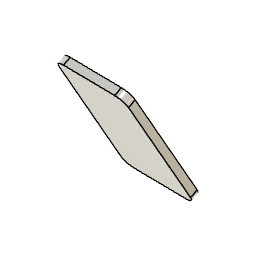
Phone Stand (Assembly) (Autodesk Fusion 360 archive; units mm, degrees)
design "Phone"
part number: 2026-06-04-19-47-22-060
Autodesk Fusion 360 part; units mm, degrees
sketch "Sketch1" plane through (0, 0, 0) normal (0, 0, 1) x (1, 0, 0)
  line L0 (0, 50) -> (-75, 50)
  line L1 (-75, 50) -> (-75, 205)
  line L2 (-75, 205) -> (0, 205)
  line L3 (0, 205) -> (0, 50)
  dimension "d1" = 75
  dimension "d2" = 155
  constraint horizontal L0
  constraint vertical L1
  constraint horizontal L2
  constraint vertical L3
  measures "d1" distance of L0.start L0.end
  measures "d2" distance of L0.start L2.end
extrude "Extrude1" add sketch "Sketch1" along normal blind 8
fillet "Fillet1" radius 10 1 edges at (0, 205, 4)
fillet "Fillet2" radius 10 1 edges at (-75, 205, 4)
fillet "Fillet3" radius 10 1 edges at (0, 50, 4)
fillet "Fillet4" radius 10 1 edges at (-75, 50, 4)
move_body "Move1" bodies 1 to x (0.996195, 0, -0.087156) y (-0.075479, 0.5, -0.86273) z (0.043578, 0.866025, 0.498097) at (214.0312, -116.6375, 222.5063)
move_body "Move2" bodies 1 to x (0.996202, -0.043268, 0.075562) y (0.043556, 0.999049, -0.002157) z (-0.075396, 0.00544, 0.997139) at (-105.4138, 10.2021, -14.7278)
move_body "Move3" bodies 1 to x (0.999848, 0.008699, -0.015111) y (-0.008687, 0.999962, 0.000826) z (0.015118, -0.000695, 0.999885) at (-2.1353, -0.3577, 0.8088)
move_body "Move4" bodies 1 to x (0.996197, 0.075622, 0.043275) y (-0.075527, 0.997136, -0.003823) z (-0.04344, 0.00054, 0.999056) at (2.0977, -3.783, -2.1098)
move_body "Move5" bodies 1 to x (0.99863, -0.045434, -0.025975) y (0.045426, 0.998967, -0.000894) z (0.025989, -0.000287, 0.999662) at (-0.665, 2.7758, 1.592)

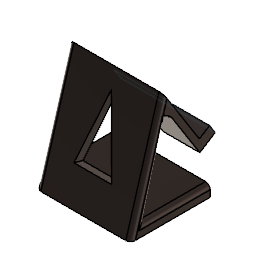
design "Phone Stand"
part number: 2026-06-02-13-47-00-270
Autodesk Fusion 360 part; units mm, degrees
sketch "Sketch1" plane through (0, 0, 0) normal (1, 0, 0) x (0, 1, 0)
  line L0 (0, 0) -> (-70, 0)
  line L1 (-70, 0) -> (-45.7841, 89.4173)
  line L2 (-45.7841, 89.4173) -> (-11.0619, 34.4149)
  line L3 (-11.0619, 34.4149) -> (5.2441, 44.7086)
  line L4 (5.2441, 44.7086) -> (-2.9089, 57.6236)
  line L5 (-2.9089, 57.6236) -> (-7.2276, 54.8973)
  line L6 (-7.2276, 54.8973) -> (-5.0683, 51.4767)
  line L7 (-5.0683, 51.4767) -> (-11.5885, 47.3606)
  line L8 (-11.5885, 47.3606) -> (-49.383, 107.2298)
  line L9 (-49.383, 107.2298) -> (-84.5009, -11.9838)
  line L10 (-84.5009, -11.9838) -> (0, -11.9838)
  line L11 (0, -11.9838) -> (0, 2.7655)
  constraint coincident L0.start origin
  constraint horizontal L0
  constraint perpendicular L2 L3
  constraint perpendicular L3 L4
  constraint perpendicular L4 L5
  constraint perpendicular L5 L6
  constraint perpendicular L4 L7
  constraint perpendicular L7 L8
  constraint horizontal L10
  constraint perpendicular L0 L11
extrude "Extrude1" add sketch "Sketch1" along normal blind 100
fillet "Fillet1" radius 2 2 edges at (50, -7.2276, 54.8973) (50, -2.9089, 57.6236)
sketch "Sketch2" plane through (0, 23.931, 15.1073) normal (0, 0.845601, 0.533815) x (-1, 0, 0)
  line L0 (0, 48.2794) -> (-100, 48.2794)
  line L1 (-100, 48.2794) -> (-100, 35.0063)
  line L2 (-100, 35.0063) -> (0, 35.0063)
  line L3 (0, 35.0063) -> (0, 48.2794)
sketch "Sketch3" plane through (0, 23.931, 15.1073) normal (0, 0.845601, 0.533815) x (-1, 0, 0)
  line L0 (-39.8663, 48.58) -> (-39.8663, 35.3379)
  line L1 (-60.2021, 48.3475) -> (-60.2021, 35)
  line L2 (-60.2021, 35) -> (-60.2021, 11.67)
  line L3 (-39.8663, 35.3379) -> (-39.8663, 11.9764)
  line L4 (-60.2021, 48.3475) -> (-39.8663, 48.58)
  line L5 (-60.2021, 11.67) -> (-39.8663, 11.9764)
  constraint vertical L1
  constraint parallel L1 L2
  constraint parallel L0 L3
extrude "Extrude2" cut sketch "Sketch3" against normal blind 25
extrude "Extrude3" cut 1 faces at (46.6221, -37.2023, 87.9346) along direction (0, 0.845601, 0.533815) blind 25
fillet "Fillet2" radius 5 2 edges at (100, -35, 0) (100, -57.8921, 44.7086)
fillet "Fillet3" radius 5 1 edges at (100, -66.942, 47.623)
fillet "Fillet4" radius 5 2 edges at (47.5, -45.7841, 89.4173) (98.2407, -46.6486, 90.7867)
fillet "Fillet5" radius 5 2 edges at (0, -66.942, 47.623) (0, -42.2504, -11.9838)
sketch "Sketch4" plane through (0, -74.5054, 21.9477) normal (0, -0.959246, 0.282574) x (1, 0, 0)
  line L0 (5, 88.9054) -> (5, -35.3731)
  line L1 (5, -35.3731) -> (95, -35.3731)
  line L2 (95, -35.3731) -> (95, 88.9054)
  line L3 (95, 88.9054) -> (5, 88.9054)
  line L4 (30, 0) -> (50, 70)
  line L5 (50, 70) -> (70, 0)
  line L6 (70, 0) -> (30, 0)
  constraint horizontal L6
extrude "Extrude4" cut sketch "Sketch4" against normal blind 110 contours L4 L5 L6
